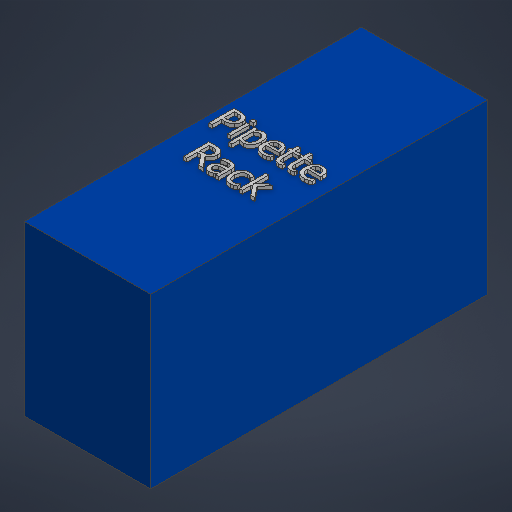
# Autodesk Inventor part: PipetteRack
Saved by Autodesk Inventor 2025.1 (Build 291241000, 241)
## iProperties
Created: 2024-10-31
Part Number: PipetteRack
Material: Generic
Document SubType Name: Modeling
Designer: jerem
Density: 1 g/cm^3
Appearance: Default
Author: jerem
Autodesk Inventor part; units mm, degrees
ref_plane "YZ Plane" through (0, 0, 0) normal (1, 0, 0) x (0, 1, 0)
ref_plane "XZ Plane" through (0, 0, 0) normal (0, 1, 0) x (-1, 0, 0)
ref_plane "XY Plane" through (0, 0, 0) normal (0, 0, 1) x (1, 0, 0)
sketch "Sketch1" plane through (0, 0, 0) normal (0, 1, 0) x (-1, 0, 0)
  line L0 (-37.5, -100) -> (37.5, -100)
  line L1 (37.5, -100) -> (37.5, 100)
  line L2 (37.5, 100) -> (-37.5, 100)
  line L3 (-37.5, 100) -> (-37.5, -100)
  line L4 (-37.5, -100) -> (37.5, 100) construction
  line L5 (37.5, -100) -> (-37.5, 100) construction
  point P0 (0, 0)
  dimension "d0" = 75
  dimension "d1" = 200
  constraints: 12 end point, 2 midpoint, 2 parallel, 1 horizontal, 1 perpendicular
  measures "d0" distance of L2.end L1.end
  measures "d1" distance of L1.end L0.end
extrude "Extrusion1" add sketch "Sketch1" along normal blind 100
sketch "Sketch2" plane through (0, 100, 0) normal (0, 1, 0) x (1, 0, 0)
  line L0 (-34.0986, 92.0661) -> (31.0676, 92.0661) construction
  line L1 (31.0676, 92.0661) -> (31.0676, -95.0971) construction
  line L2 (31.0676, -95.0971) -> (-34.0986, -95.0971) construction
  line L3 (-34.0986, -95.0971) -> (-34.0986, 92.0661) construction
  spline S0 degree 2 poles (-22.022, 13.9206) (-22.022, 12.9481) (-22.7148, 11.1977) (-23.3348, 10.5899) knots 0 0 0 1 2 2 2
  spline S1 degree 2 poles (-23.3348, 10.5899) (-24.1127, 9.8241) (-26.2157, 9.034) (-27.8202, 9.034) knots 0 0 0 1 2 2 2
  line L4 (-27.8202, 9.034) -> (-29.5098, 9.034)
  line L5 (-29.5098, 9.034) -> (-29.5098, 3.4425)
  line L6 (-29.5098, 3.4425) -> (-31.5033, 3.4425)
  line L7 (-31.5033, 3.4425) -> (-31.5033, 18.4425)
  line L8 (-31.5033, 18.4425) -> (-27.7351, 18.4425)
  spline S2 degree 2 poles (-27.7351, 18.4425) (-26.398, 18.4425) (-24.526, 18.0049) (-23.8088, 17.5065) knots 0 0 0 1 2 2 2
  spline S3 degree 2 poles (-23.8088, 17.5065) (-22.9701, 16.9352) (-22.022, 15.1726) (-22.022, 13.9206) knots 0 0 0 1 2 2 2
  spline S4 degree 2 poles (-24.1006, 13.8598) (-24.1006, 14.6378) (-24.6354, 15.7804) (-25.1824, 16.1451) knots 0 0 0 1 2 2 2
  spline S5 degree 2 poles (-25.1824, 16.1451) (-25.6565, 16.4611) (-26.9207, 16.7164) (-27.8567, 16.7164) knots 0 0 0 1 2 2 2
  line L9 (-27.8567, 16.7164) -> (-29.5098, 16.7164)
  line L10 (-29.5098, 16.7164) -> (-29.5098, 10.7358)
  line L11 (-29.5098, 10.7358) -> (-28.1484, 10.7358)
  spline S6 degree 2 poles (-28.1484, 10.7358) (-26.9328, 10.7358) (-25.4377, 11.1248) (-24.9515, 11.6353) knots 0 0 0 1 2 2 2
  spline S7 degree 2 poles (-24.9515, 11.6353) (-24.5017, 12.0851) (-24.1006, 13.1426) (-24.1006, 13.8598) knots 0 0 0 1 2 2 2
  line L12 (-18.3388, 3.4425) -> (-20.2351, 3.4425)
  line L13 (-20.2351, 3.4425) -> (-20.2351, 14.6985)
  line L14 (-20.2351, 14.6985) -> (-18.3388, 14.6985)
  line L15 (-18.3388, 14.6985) -> (-18.3388, 3.4425)
  line L16 (-18.2051, 16.5705) -> (-20.3567, 16.5705)
  line L17 (-20.3567, 16.5705) -> (-20.3567, 18.5397)
  line L18 (-20.3567, 18.5397) -> (-18.2051, 18.5397)
  line L19 (-18.2051, 18.5397) -> (-18.2051, 16.5705)
  spline S8 degree 2 poles (-6.1225, 9.3744) (-6.1225, 6.5543) (-8.8088, 3.2237) (-10.8631, 3.2237) knots 0 0 0 1 2 2 2
  spline S9 degree 2 poles (-10.8631, 3.2237) (-11.7019, 3.2237) (-12.9904, 3.6126) (-13.6589, 4.0138) knots 0 0 0 1 2 2 2
  line L20 (-13.6589, 4.0138) -> (-13.6589, -0.7026)
  line L21 (-13.6589, -0.7026) -> (-15.5552, -0.7026)
  line L22 (-15.5552, -0.7026) -> (-15.5552, 14.6985)
  line L23 (-15.5552, 14.6985) -> (-13.6589, 14.6985)
  line L24 (-13.6589, 14.6985) -> (-13.6589, 13.5194)
  spline S10 degree 2 poles (-13.6589, 13.5194) (-12.9539, 14.1637) (-11.2278, 15.0146) (-10.2189, 15.0146) knots 0 0 0 1 2 2 2
  spline S11 degree 2 poles (-10.2189, 15.0146) (-8.2862, 15.0146) (-6.1225, 11.9514) (-6.1225, 9.3744) knots 0 0 0 1 2 2 2
  spline S12 degree 2 poles (-8.0795, 9.1556) (-8.0795, 11.0883) (-9.3072, 13.2156) (-10.6808, 13.2156) knots 0 0 0 1 2 2 2
  spline S13 degree 2 poles (-10.6808, 13.2156) (-11.4831, 13.2156) (-12.9904, 12.4984) (-13.6589, 11.9392) knots 0 0 0 1 2 2 2
  line L25 (-13.6589, 11.9392) -> (-13.6589, 5.5454)
  spline S14 degree 2 poles (-13.6589, 5.5454) (-12.9174, 5.1929) (-11.8599, 4.9254) (-11.1792, 4.9254) knots 0 0 0 1 2 2 2
  spline S15 degree 2 poles (-11.1792, 4.9254) (-9.7084, 4.9254) (-8.0795, 7.0891) (-8.0795, 9.1556) knots 0 0 0 1 2 2 2
  spline S16 degree 2 poles (0.7333, 3.1872) (-1.9652, 3.1872) (-4.9312, 6.2139) (-4.9312, 9.0097) knots 0 0 0 1 2 2 2
  spline S17 degree 2 poles (-4.9312, 9.0097) (-4.9312, 11.7569) (-2.0503, 15.0146) (0.2714, 15.0146) knots 0 0 0 1 2 2 2
  spline S18 degree 2 poles (0.2714, 15.0146) (1.3168, 15.0146) (2.9335, 14.4068) (3.5291, 13.7626) knots 0 0 0 1 2 2 2
  spline S19 degree 2 poles (3.5291, 13.7626) (4.1369, 13.1183) (4.7811, 11.2585) (4.7811, 9.9092) knots 0 0 0 1 2 2 2
  line L26 (4.7811, 9.9092) -> (4.7811, 8.876)
  line L27 (4.7811, 8.876) -> (-3.0106, 8.876)
  spline S20 degree 2 poles (-3.0106, 8.876) (-3.0106, 6.919) (-1.0414, 4.8404) (0.709, 4.8404) knots 0 0 0 1 2 2 2
  spline S21 degree 2 poles (0.709, 4.8404) (1.3289, 4.8404) (2.5323, 5.1199) (3.0185, 5.3387) knots 0 0 0 1 2 2 2
  spline S22 degree 2 poles (3.0185, 5.3387) (3.5291, 5.5818) (4.2341, 6.0073) (4.4651, 6.2018) knots 0 0 0 1 2 2 2
  line L28 (4.4651, 6.2018) -> (4.5745, 6.2018)
  line L29 (4.5745, 6.2018) -> (4.5745, 4.1353)
  spline S23 degree 2 poles (4.5745, 4.1353) (4.2463, 4.0016) (3.2495, 3.6126) (2.8605, 3.5032) knots 0 0 0 1 2 2 2
  spline S24 degree 2 poles (2.8605, 3.5032) (2.3135, 3.3452) (1.414, 3.1872) (0.7333, 3.1872) knots 0 0 0 1 2 2 2
  spline S25 degree 2 poles (2.9335, 10.3225) (2.9091, 11.0883) (2.5931, 12.2066) (2.2892, 12.5835) knots 0 0 0 1 2 2 2
  spline S26 degree 2 poles (2.2892, 12.5835) (1.961, 13.0089) (0.9278, 13.4587) (0.162, 13.4587) knots 0 0 0 1 2 2 2
  spline S27 degree 2 poles (0.162, 13.4587) (-0.5917, 13.4587) (-1.6492, 13.0089) (-2.0868, 12.5713) knots 0 0 0 1 2 2 2
  spline S28 degree 2 poles (-2.0868, 12.5713) (-2.5123, 12.1216) (-2.9499, 11.0397) (-3.0106, 10.3225) knots 0 0 0 1 2 2 2
  line L30 (-3.0106, 10.3225) -> (2.9335, 10.3225)
  spline S29 degree 2 poles (10.1053, 3.2237) (8.5615, 3.2237) (6.8232, 4.9862) (6.8232, 6.8946) knots 0 0 0 1 2 2 2
  line L31 (6.8232, 6.8946) -> (6.8232, 13.1305)
  line L32 (6.8232, 13.1305) -> (5.5469, 13.1305)
  line L33 (5.5469, 13.1305) -> (5.5469, 14.6985)
  line L34 (5.5469, 14.6985) -> (6.8232, 14.6985)
  line L35 (6.8232, 14.6985) -> (6.8232, 17.9319)
  line L36 (6.8232, 17.9319) -> (8.7195, 17.9319)
  line L37 (8.7195, 17.9319) -> (8.7195, 14.6985)
  line L38 (8.7195, 14.6985) -> (12.2082, 14.6985)
  line L39 (12.2082, 14.6985) -> (12.2082, 13.1305)
  line L40 (12.2082, 13.1305) -> (8.7195, 13.1305)
  line L41 (8.7195, 13.1305) -> (8.7195, 7.7699)
  spline S30 degree 2 poles (8.7195, 7.7699) (8.7195, 6.919) (8.7803, 5.983) (8.9869, 5.5818) knots 0 0 0 1 2 2 2
  spline S31 degree 2 poles (8.9869, 5.5818) (9.1571, 5.2293) (9.9229, 4.8768) (10.5793, 4.8768) knots 0 0 0 1 2 2 2
  spline S32 degree 2 poles (10.5793, 4.8768) (11.0412, 4.8768) (11.9043, 5.1564) (12.0988, 5.2415) knots 0 0 0 1 2 2 2
  line L42 (12.0988, 5.2415) -> (12.2082, 5.2415)
  line L43 (12.2082, 5.2415) -> (12.2082, 3.5397)
  spline S33 degree 2 poles (12.2082, 3.5397) (11.6733, 3.3938) (10.5793, 3.2237) (10.1053, 3.2237) knots 0 0 0 1 2 2 2
  spline S34 degree 2 poles (17.0096, 3.2237) (15.4659, 3.2237) (13.7276, 4.9862) (13.7276, 6.8946) knots 0 0 0 1 2 2 2
  line L44 (13.7276, 6.8946) -> (13.7276, 13.1305)
  line L45 (13.7276, 13.1305) -> (12.4513, 13.1305)
  line L46 (12.4513, 13.1305) -> (12.4513, 14.6985)
  line L47 (12.4513, 14.6985) -> (13.7276, 14.6985)
  line L48 (13.7276, 14.6985) -> (13.7276, 17.9319)
  line L49 (13.7276, 17.9319) -> (15.6239, 17.9319)
  line L50 (15.6239, 17.9319) -> (15.6239, 14.6985)
  line L51 (15.6239, 14.6985) -> (19.1125, 14.6985)
  line L52 (19.1125, 14.6985) -> (19.1125, 13.1305)
  line L53 (19.1125, 13.1305) -> (15.6239, 13.1305)
  line L54 (15.6239, 13.1305) -> (15.6239, 7.7699)
  spline S35 degree 2 poles (15.6239, 7.7699) (15.6239, 6.919) (15.6847, 5.983) (15.8913, 5.5818) knots 0 0 0 1 2 2 2
  spline S36 degree 2 poles (15.8913, 5.5818) (16.0615, 5.2293) (16.8273, 4.8768) (17.4837, 4.8768) knots 0 0 0 1 2 2 2
  spline S37 degree 2 poles (17.4837, 4.8768) (17.9456, 4.8768) (18.8087, 5.1564) (19.0031, 5.2415) knots 0 0 0 1 2 2 2
  line L55 (19.0031, 5.2415) -> (19.1125, 5.2415)
  line L56 (19.1125, 5.2415) -> (19.1125, 3.5397)
  spline S38 degree 2 poles (19.1125, 3.5397) (18.5777, 3.3938) (17.4837, 3.2237) (17.0096, 3.2237) knots 0 0 0 1 2 2 2
  spline S39 degree 2 poles (25.397, 3.1872) (22.6984, 3.1872) (19.7325, 6.2139) (19.7325, 9.0097) knots 0 0 0 1 2 2 2
  spline S40 degree 2 poles (19.7325, 9.0097) (19.7325, 11.7569) (22.6134, 15.0146) (24.9351, 15.0146) knots 0 0 0 1 2 2 2
  spline S41 degree 2 poles (24.9351, 15.0146) (25.9805, 15.0146) (27.5971, 14.4068) (28.1928, 13.7626) knots 0 0 0 1 2 2 2
  spline S42 degree 2 poles (28.1928, 13.7626) (28.8006, 13.1183) (29.4448, 11.2585) (29.4448, 9.9092) knots 0 0 0 1 2 2 2
  line L57 (29.4448, 9.9092) -> (29.4448, 8.876)
  line L58 (29.4448, 8.876) -> (21.6531, 8.876)
  spline S43 degree 2 poles (21.6531, 8.876) (21.6531, 6.919) (23.6223, 4.8404) (25.3727, 4.8404) knots 0 0 0 1 2 2 2
  spline S44 degree 2 poles (25.3727, 4.8404) (25.9926, 4.8404) (27.196, 5.1199) (27.6822, 5.3387) knots 0 0 0 1 2 2 2
  spline S45 degree 2 poles (27.6822, 5.3387) (28.1928, 5.5818) (28.8978, 6.0073) (29.1288, 6.2018) knots 0 0 0 1 2 2 2
  line L59 (29.1288, 6.2018) -> (29.2382, 6.2018)
  line L60 (29.2382, 6.2018) -> (29.2382, 4.1353)
  spline S46 degree 2 poles (29.2382, 4.1353) (28.91, 4.0016) (27.9132, 3.6126) (27.5242, 3.5032) knots 0 0 0 1 2 2 2
  spline S47 degree 2 poles (27.5242, 3.5032) (26.9772, 3.3452) (26.0777, 3.1872) (25.397, 3.1872) knots 0 0 0 1 2 2 2
  spline S48 degree 2 poles (27.5971, 10.3225) (27.5728, 11.0883) (27.2568, 12.2066) (26.9529, 12.5835) knots 0 0 0 1 2 2 2
  spline S49 degree 2 poles (26.9529, 12.5835) (26.6247, 13.0089) (25.5915, 13.4587) (24.8257, 13.4587) knots 0 0 0 1 2 2 2
  spline S50 degree 2 poles (24.8257, 13.4587) (24.072, 13.4587) (23.0145, 13.0089) (22.5769, 12.5713) knots 0 0 0 1 2 2 2
  spline S51 degree 2 poles (22.5769, 12.5713) (22.1514, 12.1216) (21.7138, 11.0397) (21.6531, 10.3225) knots 0 0 0 1 2 2 2
  line L61 (21.6531, 10.3225) -> (27.5971, 10.3225)
  line L62 (-10.0973, -21.2546) -> (-12.6865, -21.2546)
  line L63 (-12.6865, -21.2546) -> (-17.4272, -15.2862)
  line L64 (-17.4272, -15.2862) -> (-19.7124, -15.2862)
  line L65 (-19.7124, -15.2862) -> (-19.7124, -21.2546)
  line L66 (-19.7124, -21.2546) -> (-21.7059, -21.2546)
  line L67 (-21.7059, -21.2546) -> (-21.7059, -6.2546)
  line L68 (-21.7059, -6.2546) -> (-17.8405, -6.2546)
  spline S52 degree 2 poles (-17.8405, -6.2546) (-16.552, -6.2546) (-14.8137, -6.5342) (-14.0236, -7.0448) knots 0 0 0 1 2 2 2
  spline S53 degree 2 poles (-14.0236, -7.0448) (-13.2335, -7.5553) (-12.3218, -9.1477) (-12.3218, -10.3268) knots 0 0 0 1 2 2 2
  spline S54 degree 2 poles (-12.3218, -10.3268) (-12.3218, -11.9678) (-13.9993, -14.1922) (-15.4336, -14.7271) knots 0 0 0 1 2 2 2
  line L69 (-15.4336, -14.7271) -> (-10.0973, -21.2546)
  spline S55 degree 2 poles (-14.4004, -10.4848) (-14.4004, -9.8284) (-14.8623, -8.8195) (-15.3486, -8.4913) knots 0 0 0 1 2 2 2
  spline S56 degree 2 poles (-15.3486, -8.4913) (-15.774, -8.2117) (-16.9045, -7.9807) (-17.7311, -7.9807) knots 0 0 0 1 2 2 2
  line L70 (-17.7311, -7.9807) -> (-19.7124, -7.9807)
  line L71 (-19.7124, -7.9807) -> (-19.7124, -13.6209)
  line L72 (-19.7124, -13.6209) -> (-17.962, -13.6209)
  spline S57 degree 2 poles (-17.962, -13.6209) (-17.099, -13.6209) (-15.7254, -13.317) (-15.2513, -12.843) knots 0 0 0 1 2 2 2
  spline S58 degree 2 poles (-15.2513, -12.843) (-14.8137, -12.4297) (-14.4004, -11.2627) (-14.4004, -10.4848) knots 0 0 0 1 2 2 2
  spline S59 degree 2 poles (-2.7797, -20.0634) (-3.0106, -20.2336) (-3.7886, -20.8414) (-4.1533, -21.0237) knots 0 0 0 1 2 2 2
  spline S60 degree 2 poles (-4.1533, -21.0237) (-4.6516, -21.2911) (-5.5876, -21.5707) (-6.4385, -21.5707) knots 0 0 0 1 2 2 2
  spline S61 degree 2 poles (-6.4385, -21.5707) (-7.1314, -21.5707) (-8.3834, -21.048) (-8.8575, -20.5739) knots 0 0 0 1 2 2 2
  spline S62 degree 2 poles (-8.8575, -20.5739) (-9.3072, -20.112) (-9.8542, -18.7506) (-9.8542, -17.9969) knots 0 0 0 1 2 2 2
  spline S63 degree 2 poles (-9.8542, -17.9969) (-9.8542, -16.83) (-8.8696, -15.1768) (-7.7999, -14.7028) knots 0 0 0 1 2 2 2
  spline S64 degree 2 poles (-7.7999, -14.7028) (-6.8518, -14.2652) (-4.2748, -13.937) (-2.7797, -13.8519) knots 0 0 0 1 2 2 2
  line L73 (-2.7797, -13.8519) -> (-2.7797, -13.4872)
  spline S65 degree 2 poles (-2.7797, -13.4872) (-2.7797, -12.8308) (-3.1808, -12.0164) (-3.5455, -11.7854) knots 0 0 0 1 2 2 2
  spline S66 degree 2 poles (-3.5455, -11.7854) (-3.9101, -11.5545) (-4.9555, -11.4086) (-5.5147, -11.4086) knots 0 0 0 1 2 2 2
  spline S67 degree 2 poles (-5.5147, -11.4086) (-6.1711, -11.4086) (-7.9458, -11.7976) (-8.8332, -12.1744) knots 0 0 0 1 2 2 2
  line L74 (-8.8332, -12.1744) -> (-8.9426, -12.1744)
  line L75 (-8.9426, -12.1744) -> (-8.9426, -10.2417)
  spline S68 degree 2 poles (-8.9426, -10.2417) (-8.4199, -10.0958) (-6.4628, -9.7311) (-5.5025, -9.7311) knots 0 0 0 1 2 2 2
  spline S69 degree 2 poles (-5.5025, -9.7311) (-4.3356, -9.7311) (-2.7432, -10.0958) (-2.1111, -10.5699) knots 0 0 0 1 2 2 2
  spline S70 degree 2 poles (-2.1111, -10.5699) (-1.4912, -11.0318) (-0.8834, -12.5026) (-0.8834, -13.5602) knots 0 0 0 1 2 2 2
  line L76 (-0.8834, -13.5602) -> (-0.8834, -21.2546)
  line L77 (-0.8834, -21.2546) -> (-2.7797, -21.2546)
  line L78 (-2.7797, -21.2546) -> (-2.7797, -20.0634)
  line L79 (-2.7797, -18.4832) -> (-2.7797, -15.3592)
  spline S71 degree 2 poles (-2.7797, -15.3592) (-3.4604, -15.42) (-5.5147, -15.6266) (-6.1589, -15.8211) knots 0 0 0 1 2 2 2
  spline S72 degree 2 poles (-6.1589, -15.8211) (-6.9126, -16.0521) (-7.8972, -17.0123) (-7.8972, -17.8632) knots 0 0 0 1 2 2 2
  spline S73 degree 2 poles (-7.8972, -17.8632) (-7.8972, -18.8357) (-6.8032, -19.8203) (-5.7578, -19.8203) knots 0 0 0 1 2 2 2
  spline S74 degree 2 poles (-5.7578, -19.8203) (-4.8704, -19.8203) (-3.4118, -19.0545) (-2.7797, -18.4832) knots 0 0 0 1 2 2 2
  spline S75 degree 2 poles (6.2519, -21.5099) (5.085, -21.5099) (3.1523, -20.7927) (2.4594, -20.0634) knots 0 0 0 1 2 2 2
  spline S76 degree 2 poles (2.4594, -20.0634) (1.7665, -19.3462) (1.0007, -17.1339) (1.0007, -15.6509) knots 0 0 0 1 2 2 2
  spline S77 degree 2 poles (1.0007, -15.6509) (1.0007, -14.1679) (1.7908, -12.0042) (2.4594, -11.2749) knots 0 0 0 1 2 2 2
  spline S78 degree 2 poles (2.4594, -11.2749) (3.1279, -10.5334) (5.1093, -9.7433) (6.2519, -9.7433) knots 0 0 0 1 2 2 2
  spline S79 degree 2 poles (6.2519, -9.7433) (7.1758, -9.7433) (8.9018, -10.266) (9.5704, -10.6063) knots 0 0 0 1 2 2 2
  line L80 (9.5704, -10.6063) -> (9.5704, -12.7336)
  line L81 (9.5704, -12.7336) -> (9.461, -12.7336)
  spline S80 degree 2 poles (9.461, -12.7336) (9.2544, -12.5634) (8.6223, -12.1258) (8.1725, -11.8948) knots 0 0 0 1 2 2 2
  spline S81 degree 2 poles (8.1725, -11.8948) (7.7714, -11.7003) (6.7017, -11.3965) (6.2155, -11.3965) knots 0 0 0 1 2 2 2
  spline S82 degree 2 poles (6.2155, -11.3965) (4.7446, -11.3965) (2.9578, -13.6209) (2.9578, -15.6509) knots 0 0 0 1 2 2 2
  spline S83 degree 2 poles (2.9578, -15.6509) (2.9578, -17.6323) (4.6839, -19.8568) (6.2155, -19.8568) knots 0 0 0 1 2 2 2
  spline S84 degree 2 poles (6.2155, -19.8568) (7.1393, -19.8568) (8.8168, -19.0909) (9.461, -18.4953) knots 0 0 0 1 2 2 2
  line L82 (9.461, -18.4953) -> (9.5704, -18.4953)
  line L83 (9.5704, -18.4953) -> (9.5704, -20.6226)
  spline S85 degree 2 poles (9.5704, -20.6226) (9.2908, -20.7563) (8.4399, -21.1331) (8.0996, -21.2182) knots 0 0 0 1 2 2 2
  spline S86 degree 2 poles (8.0996, -21.2182) (7.6134, -21.364) (6.8476, -21.5099) (6.2519, -21.5099) knots 0 0 0 1 2 2 2
  line L84 (20.6198, -21.2546) -> (18.1279, -21.2546)
  line L85 (18.1279, -21.2546) -> (13.9464, -15.8211)
  line L86 (13.9464, -15.8211) -> (13.1928, -16.5504)
  line L87 (13.1928, -16.5504) -> (13.1928, -21.2546)
  line L88 (13.1928, -21.2546) -> (11.2965, -21.2546)
  line L89 (11.2965, -21.2546) -> (11.2965, -5.5861)
  line L90 (11.2965, -5.5861) -> (13.1928, -5.5861)
  line L91 (13.1928, -5.5861) -> (13.1928, -14.7514)
  line L92 (13.1928, -14.7514) -> (17.6417, -9.9986)
  line L93 (17.6417, -9.9986) -> (19.9999, -9.9986)
  line L94 (19.9999, -9.9986) -> (15.3808, -14.7028)
  line L95 (15.3808, -14.7028) -> (20.6198, -21.2546)
  point P0 (0, 0)
  constraints: 2 other
extrude "Extrusion2" add sketch "Sketch2" along normal blind 2
body "Solid1"
